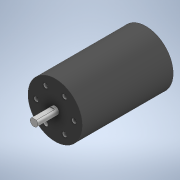
# Autodesk Inventor part: silnik 3660
Saved by Autodesk Inventor 2021 (Build 250183000, 183)
## iProperties
Created: 2021-06-24
Part Number: silnik 3660
Material: Generic
Document SubType Name: Modeling
Designer: Łukasz
Density: 1 g/cm^3
Appearance: Default
Author: Łukasz
Autodesk Inventor part; units mm, degrees
ref_plane "YZ Plane" through (0, 0, 0) normal (1, 0, 0) x (0, 1, 0)
ref_plane "XZ Plane" through (0, 0, 0) normal (0, 1, 0) x (-1, 0, 0)
ref_plane "XY Plane" through (0, 0, 0) normal (0, 0, 1) x (1, 0, 0)
sketch "Sketch1" plane through (0, 0, 0) normal (0, 0, 1) x (1, 0, 0)
  circle A0 centre (0, 0) radius 18
  dimension "d0" = 36
  constraints: 1 centre point, 1 coincident
  measures "d0" diameter of A0
extrude "Extrusion1" add sketch "Sketch1" along normal blind 60
sketch "Sketch2" plane through (0, 0, 60) normal (0, 0, 1) x (1, 0, 0)
  circle A0 centre (0, 0) radius 2.5
  dimension "d3" = 5
  constraints: 1 centre point, 1 coincident
  measures "d3" diameter of A0
extrude "Extrusion2" add sketch "Sketch2" along normal blind 14
sketch "Sketch3" plane through (0, 0, 74) normal (0, 0, 1) x (1, 0, 0)
  circle A0 centre (0, 0) radius 2.5 projected
  line L0 (-1.5, 2) -> (1.5, 2)
  dimension "d6" = 4.5
  constraints: 2 end point, 2 point on circle, 1 horizontal
extrude "Extrusion3" cut sketch "Sketch3" against normal blind 12 contours L0 A0 picked at (-0.3466, 2.0912)
sketch "Sketch4" plane through (0, 0, 60) normal (0, 0, 1) x (1, 0, 0)
  circle A0 centre (-12.5, 0) radius 1.5
  circle A1 centre (0, 0) radius 18 projected
  circle A2 centre (-6.25, -10.8253) radius 1.5
  circle A3 centre (6.25, -10.8253) radius 1.5
  circle A4 centre (12.5, 0) radius 1.5
  circle A5 centre (6.25, 10.8253) radius 1.5
  circle A6 centre (-6.25, 10.8253) radius 1.5
  dimension "d9" = 3
  dimension "d10" = 12.5
  dimension "d13" = 360
  constraints: 6 centre point, 13 other
  measures "d9" diameter of A0
  measures "d10" distance of A1.centre A0.centre
extrude "Extrusion4" cut sketch "Sketch4" against normal blind 10 contours A0 | A2 | A3 | A4 | A5 | A6
body "Solid1"
